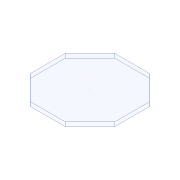
# Autodesk Inventor part: Substrate
Saved by Autodesk Inventor 2020 (Build 240168000, 168)
## iProperties
Created: 2022-03-01
Part Number: Substrate
Material: Generic
Document SubType Name: Modeling
Designer: ferrerx
Density: 1 g/cm^3
Appearance: Clear - Blue
Author: ferrerx
Autodesk Inventor part; units mm, degrees
ref_plane "YZ Plane" through (0, 0, 0) normal (1, 0, 0) x (0, 1, 0)
ref_plane "XZ Plane" through (0, 0, 0) normal (0, 1, 0) x (-1, 0, 0)
ref_plane "XY Plane" through (0, 0, 0) normal (0, 0, 1) x (1, 0, 0)
sketch "Sketch1" plane through (0, 0, 0) normal (0, 1, 0) x (-1, 0, 0)
  line L0 (0, -5.2573) -> (-3.0902, -4.2533) construction
  line L1 (-3.0902, -4.2533) -> (-5, -1.6246) construction
  line L2 (-5, -1.6246) -> (-5, 1.6246) construction
  line L3 (-5, 1.6246) -> (-3.0902, 4.2533) construction
  line L4 (-3.0902, 4.2533) -> (0, 5.2573) construction
  line L5 (0, 5.2573) -> (3.0902, 4.2533) construction
  line L6 (3.0902, 4.2533) -> (5, 1.6246) construction
  line L7 (5, 1.6246) -> (5, -1.6246) construction
  line L8 (5, -1.6246) -> (3.0902, -4.2533) construction
  line L9 (3.0902, -4.2533) -> (0, -5.2573) construction
  line L10 (-2.0711, -5) -> (-5, -2.0711)
  line L11 (-5, -2.0711) -> (-5, 2.0711)
  line L12 (-5, 2.0711) -> (-2.0711, 5)
  line L13 (-2.0711, 5) -> (2.0711, 5)
  line L14 (2.0711, 5) -> (5, 2.0711)
  line L15 (5, 2.0711) -> (5, -2.0711)
  line L16 (5, -2.0711) -> (2.0711, -5)
  line L17 (2.0711, -5) -> (-2.0711, -5)
  line L18 (0, 0) -> (-10.1721, 0) construction
  dimension "d0" = 10
  dimension "d3" = 10
  constraints: 38 end point, 2 coincident, 1 horizontal, 1 parallel, 38 other
  measures "d0" distance between parallel lines of L2 L7
  measures "d3" distance between parallel lines of L13 L17
extrude "Extrusion1" add sketch "Sketch1" along normal blind 0.5
body "Solid1"
